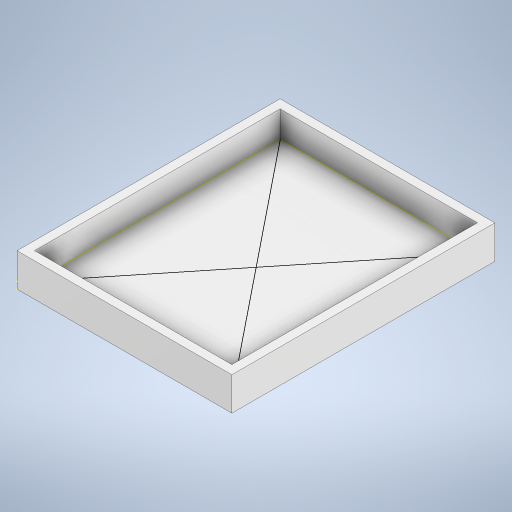
# Autodesk Inventor part: Case_3d_model
Saved by Autodesk Inventor 2023 (Build 270158000, 158)
## iProperties
Created: 2023-03-21
Part Number: Case_3d_model
Material: ABS Plastic
Document SubType Name: Sheet Metal
Designer: Inteli
Density: 1.06 g/cm^3
Sheet Metal Rule: Default
Appearance: Smooth - White
Author: Inteli
Autodesk Inventor part; units mm, degrees
ref_plane "YZ Plane" through (0, 0, 0) normal (1, 0, 0) x (0, 1, 0)
ref_plane "XZ Plane" through (0, 0, 0) normal (0, 1, 0) x (-1, 0, 0)
ref_plane "XY Plane" through (0, 0, 0) normal (0, 0, 1) x (1, 0, 0)
sketch "Sketch1" plane through (0, 0, 0) normal (0, 1, 0) x (-1, 0, 0)
  line L0 (0, 0) -> (0, -250)
  line L1 (-200, 0) -> (0, 0)
  line L2 (0, -250) -> (0, -300)
  line L3 (0, -300) -> (-200, -300)
  line L4 (-200, -300) -> (-230, -300)
  line L5 (-230, 0) -> (-200, 0)
  line L6 (-230, -300) -> (-245, -300)
  line L7 (-245, -300) -> (-245, 0)
  line L8 (-245, 0) -> (-230, 0)
  dimension "d0" = 250
  dimension "d4" = 50
  dimension "d12" = 30
  dimension "d24" = 15
  constraints: 18 end point, 2 horizontal, 2 perpendicular, 2 vertical
  measures "d0" distance of L0.start L0.end
  measures "d4" distance of L0.end L2.end
  measures "d12" distance of L3.end L4.end
  measures "d24" distance of L4.end L6.end
extrude "Extrusion1" add sketch "Sketch1" along normal blind 38
sketch "Sketch2" plane through (0, 38, 0) normal (0, 1, 0) x (1, 0, 0)
  line L0 (0, 300) -> (0, 0) projected
  line L1 (0, 0) -> (245, 0) projected
  line L2 (10, 10) -> (10, 290)
  line L3 (245, 300) -> (0, 300) projected
  line L4 (245, 0) -> (245, 300) projected
  line L5 (245, 290) -> (235, 290)
  line L6 (235, 290) -> (235, 10)
  line L7 (235, 290) -> (10, 290)
  line L8 (0, 300) -> (0, 0) projected
  line L9 (235, 10) -> (10, 10)
  dimension "d25" = 10
  constraints: 10 end point, 2 perpendicular, 1 point on line
  measures "d25" distance of L5.end L5.start
extrude "Extrusion2" cut sketch "Sketch2" against normal blind 30 contours L2 L7 L6 L9
sketch "Sketch3" plane through (0, 0, 0) normal (0, 0, 1) x (1, 0, 0)
  point P0 (0, 0)
  point P1 (114.7739, 18.6848)
hole "Hole1" at (114.7739, 18.6848, 0) direction (0, 0, 1) diameter 30 end through all
sketch "Sketch4" plane through (230, 0, 0) normal (1, 0, 0) x (0, 0, -1)
  line L0 (0, 0) -> (0, 38) projected
  line L1 (300, 0) -> (300, 38) projected
  circle A0 centre (150, 23.0148) radius 13.5
  dimension "d21" = 27
  constraints: 1 centre point
  measures "d21" diameter of A0
extrude "Extrusion3" [suppressed]
sketch "Sketch5" plane through (0, 0, 0) normal (0, -1, 0) x (1, 0, 0)
  point P0 (0, 0)
sketch "Sketch6" plane through (0, 8, 0) normal (0, 1, 0) x (1, 0, 0)
  point P0 (0, 0)
sketch "Sketch7" plane through (0, 8, 0) normal (0, 1, 0) x (1, 0, 0)
  line L0 (10, 290) -> (235, 290) projected
  line L1 (235, 10) -> (10, 10) projected
  line L2 (235, 290) -> (10, 10)
  line L3 (10, 10) -> (10, 290) projected
  line L4 (235, 10) -> (10, 290)
  point P0 (0, 0)
  constraints: 4 end point
equation "\"d19\" = Thickness"
equation "\"BendRadius\" = Thickness"
equation "\"BendReliefWidth\" = Thickness"
equation "\"BendReliefDepth\" = 0.5 * Thickness"
equation "\"CornerReliefSize\" = 4 * Thickness"
equation "\"MinimumRemnant\" = 2 * Thickness"
equation "\"TransitionRadius\" = BendRadius"
equation "\"JacobiRadiusSize\" = BendRadius"
equation "\"GapSize\" = Thickness"
equation "\"Thickness\" = 3.048"
body "Solid1"
